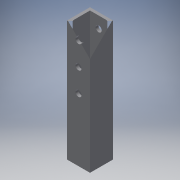
# Autodesk Inventor part: upright beam
Saved by Autodesk Inventor 2016 (Build 200138000, 138)
## iProperties
Created: 2016-04-20
Part Number: upright beam
Material: Generic
Document SubType Name: Modeling
Designer: gus
Density: 1 g/cm^3
Appearance: Default
Author: gus
Autodesk Inventor part; units mm, degrees
ref_plane "YZ Plane" through (0, 0, 0) normal (1, 0, 0) x (0, 1, 0)
ref_plane "XZ Plane" through (0, 0, 0) normal (0, 1, 0) x (-1, 0, 0)
ref_plane "XY Plane" through (0, 0, 0) normal (0, 0, 1) x (1, 0, 0)
sketch "Sketch1" plane through (0, 0, 0) normal (0, 1, 0) x (-1, 0, 0)
  line L0 (0, 0) -> (-25.4, 0)
  line L1 (-25.4, 0) -> (-25.4, 25.4)
  line L2 (-25.4, 25.4) -> (0, 25.4)
  line L3 (0, 25.4) -> (0, 0)
  line L4 (-22.225, 22.225) -> (-22.225, 3.175)
  line L5 (-22.225, 3.175) -> (-3.175, 3.175)
  line L6 (-3.175, 3.175) -> (-3.175, 22.225)
  line L7 (-3.175, 22.225) -> (-22.225, 22.225)
  dimension "d0" = 25.4
  dimension "d1" = 25.4
  dimension "d2" = 3.175
  constraints: 16 end point, 4 parallel, 2 perpendicular, 1 horizontal, 3 other
  measures "d0" distance of L1.end L2.end
  measures "d1" distance of L0.end L1.end
  measures "d2" distance between parallel lines of L1 L4
extrude "Extrusion1" add sketch "Sketch1" along normal blind 107.8738
sketch "Sketch2" plane through (0, 0, 25.4) normal (0, 0, 1) x (1, 0, 0)
  circle A0 centre (12.7, 95.1738) radius 3.3734
  line L0 (25.4, 0) -> (25.4, 107.8738) projected
  line L1 (0, 107.8738) -> (25.4, 107.8738) projected
  circle A1 centre (12.7, 69.7738) radius 3.3734
  circle A2 centre (12.7, 44.3738) radius 3.3734
  point P0 (0, 0)
  dimension "d5" = 6.7469
  dimension "d6" = 12.7
  dimension "d7" = 12.7
  dimension "d8" = 6.7469
  dimension "d9" = 12.7
  dimension "d10" = 25.4
  dimension "d11" = 6.7469
  dimension "d12" = 25.4
  dimension "d13" = 12.7
  constraints: 3 centre point
  measures "d5" diameter of A0
  measures "d6" distance from line of L0 A0.centre
  measures "d7" distance from line of L1 A0.centre
  measures "d8" diameter of A1
  measures "d9" distance from line of L0 A1.centre
  measures "d10" distance of A0.centre A1.centre
  measures "d11" diameter of A2
  measures "d12" distance of A2.centre A1.centre
  measures "d13" distance from line of L0 A2.centre
extrude "Extrusion2" cut sketch "Sketch2" against normal blind 25.4
sketch "Sketch3" plane through (0, 0, 0) normal (-1, 0, 0) x (0, 0, 1)
  circle A0 centre (12.7, 12.7) radius 3.3734
  circle A1 centre (12.7, 38.1) radius 3.3734
  line L0 (25.4, 0) -> (25.4, 107.8738) projected
  line L1 (25.4, 0) -> (0, 0) projected
  dimension "d16" = 6.7469
  dimension "d17" = 12.7
  dimension "d18" = 12.7
  dimension "d19" = 12.7
  dimension "d20" = 38.1
  constraints: 2 centre point, 1 equal radius
  measures "d16" diameter of A0
  measures "d17" distance from line of L0 A1.centre
  measures "d18" distance from line of A0.centre L0
  measures "d19" distance from line of L1 A0.centre
  measures "d20" distance from line of L1 A1.centre
extrude "Extrusion3" cut sketch "Sketch3" against normal blind 25.4
body "Solid1"
